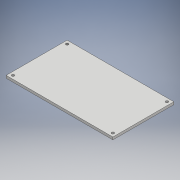
# Autodesk Inventor part: 基本板上
Saved by Autodesk Inventor 2017 (Build 210142000, 142)
## iProperties
Part Number: 基本板上
Material: 一般
Document SubType Name: Modeling
Designer: HISAAKI
Density: 1 g/cm^3
Appearance: 既定
Author: HISAAKI
Autodesk Inventor part; units mm, degrees
ref_plane "YZ Plane" through (0, 0, 0) normal (1, 0, 0) x (0, 1, 0)
ref_plane "XZ Plane" through (0, 0, 0) normal (0, 1, 0) x (-1, 0, 0)
ref_plane "XY Plane" through (0, 0, 0) normal (0, 0, 1) x (1, 0, 0)
sketch "スケッチ1" plane through (0, 0, 0) normal (0, 0, 1) x (1, 0, 0)
  line L0 (0, 0) -> (140, 0)
  line L1 (140, 0) -> (140, 80)
  line L2 (140, 80) -> (0, 80)
  line L3 (0, 80) -> (0, 0)
  dimension "d0" = 140
  dimension "d1" = 80
  constraints: 8 end point, 2 parallel, 1 horizontal, 1 perpendicular
  measures "d0" distance of L2.end L1.end
  measures "d1" distance of L1.end L0.end
extrude "押し出し1" add sketch "スケッチ1" along normal blind 3.3
hole "穴1" at (4.5, 4.5, 3.3) direction (0, 0, -1) diameter 3.4 end through all
hole "穴2" at (4.5, 75.5, 3.3) direction (0, 0, -1) diameter 3.4 end through all
hole "穴3" at (135.5, 4.5, 3.3) direction (0, 0, -1) diameter 3.4 end through all
hole "穴4" at (135.5, 75.5, 3.3) direction (0, 0, -1) diameter 3.4 end through all
